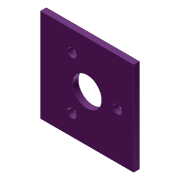
# Autodesk Inventor part: BearingRetainerPlate
Saved by Autodesk Inventor 2012 (Build 160160000, 160)
## iProperties
Created: 2012-11-16
Part Number: BearingRetainerPlate
Material: Aluminum-6061
Document SubType Name: Modeling
Designer: JesseK
Mass: 20.0192 g
Surface Area: 56.0278 cm^2
Volume: 7.38718 cm^3
Density: 2.71 g/cm^3
Author: JesseK
Autodesk Inventor part; units mm, degrees
ref_plane "YZ Plane" through (0, 0, 0) normal (1, 0, 0) x (0, 1, 0)
ref_plane "XZ Plane" through (0, 0, 0) normal (0, 1, 0) x (-1, 0, 0)
ref_plane "XY Plane" through (0, 0, 0) normal (0, 0, 1) x (1, 0, 0)
sketch "Sketch1" plane through (0, 0, 0) normal (0, 0, 1) x (1, 0, 0)
  circle A0 centre (0, 0) radius 7.9375
  line L0 (-25.4, 25.4) -> (25.4, 25.4)
  line L1 (25.4, 25.4) -> (25.4, -25.4)
  line L2 (25.4, -25.4) -> (-25.4, -25.4)
  line L3 (-25.4, -25.4) -> (-25.4, 25.4)
  line L4 (-25.4, 25.4) -> (0, 0) construction
  line L5 (0, 0) -> (25.4, 25.4) construction
  line L6 (8.2489, 14.2875) -> (16.4978, 0) construction
  line L7 (16.4978, 0) -> (8.2489, -14.2875) construction
  line L8 (8.2489, -14.2875) -> (-8.2489, -14.2875) construction
  line L9 (-8.2489, -14.2875) -> (-16.4978, 0) construction
  line L10 (-16.4978, 0) -> (-8.2489, 14.2875) construction
  line L11 (-8.2489, 14.2875) -> (8.2489, 14.2875) construction
  circle A1 centre (-8.2489, 14.2875) radius 2.4384
  circle A2 centre (16.4978, 0) radius 2.4384
  circle A3 centre (-8.2489, -14.2875) radius 2.4384
  line L12 (0, 0) -> (-25.4, -25.4) construction
  line L13 (0, 0) -> (25.4, -25.4) construction
  dimension "d0" = 50.8
  dimension "d1" = 28.575
  dimension "d2" = 15.875
  dimension "d3" = 4.8768
  constraints: 28 end point, 5 coincident, 4 centre point, 4 perpendicular, 2 equal radius, 2 horizontal, 2 parallel, 13 other
  measures "d0" distance of L0.start L0.end
  measures "d1" distance between parallel lines of L8 L11
  measures "d2" diameter of A0
  measures "d3" diameter of A1
extrude "Extrusion1" add sketch "Sketch1" along normal blind 3.175
body "Solid1"
